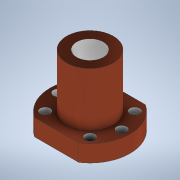
# Autodesk Inventor part: Tuerca 16
Saved by Autodesk Inventor 2021 (Build 250183000, 183)
## iProperties
Created: 2022-01-20
Part Number: Tuerca 16
Material: Generic
Document SubType Name: Modeling
Designer: deuts
Density: 1 g/cm^3
Appearance: Default
Author: deuts
Autodesk Inventor part; units mm, degrees
ref_plane "YZ Plane" through (0, 0, 0) normal (1, 0, 0) x (0, 1, 0)
ref_plane "XZ Plane" through (0, 0, 0) normal (0, 1, 0) x (-1, 0, 0)
ref_plane "XY Plane" through (0, 0, 0) normal (0, 0, 1) x (1, 0, 0)
sketch "Sketch1" plane through (0, 0, 0) normal (0, 1, 0) x (-1, 0, 0)
  line L0 (-13.2665, 20) -> (13.2665, 20)
  line L1 (13.2665, -20) -> (-13.2665, -20)
  arc A0 (13.2665, -20) -> (13.2665, 20) centre (0, 0) ccw
  arc A1 (-13.2665, 20) -> (-13.2665, -20) centre (0, 0) ccw
  circle A2 centre (19, 0) radius 3
  circle A3 centre (13.435, 13.435) radius 3
  circle A4 centre (13.435, -13.435) radius 3
  line L2 (0, 0) -> (-19, 0)
  circle A5 centre (-19, 0) radius 3
  circle A6 centre (-13.435, -13.435) radius 3
  circle A7 centre (-13.435, 13.435) radius 3
  dimension "d2" = 40
  dimension "d7" = 45
  dimension "d11" = 45
  dimension "d17" = 45
  dimension "d21" = 45
  constraints: 8 centre point, 6 end point, 4 point on circle, 2 coincident, 2 horizontal, 1 parallel, 12 other
  measures "d2" distance between parallel lines of L1 L0
extrude "Extrusion1" add sketch "Sketch1" along normal blind 10
sketch "Sketch2" plane through (0, 10, 0) normal (0, 1, 0) x (1, 0, 0)
  circle A0 centre (0, 0) radius 14
  dimension "d25" = 28
  constraints: 1 centre point, 1 coincident
  measures "d25" diameter of A0
extrude "Extrusion2" add sketch "Sketch2" along normal blind 32
sketch "Sketch3" plane through (0, 42, 0) normal (0, 1, 0) x (1, 0, 0)
  point P0 (0, 0)
  point P1 (0, 0)
  constraints: 1 coincident
hole "Hole1" at (0, 42, 0) direction (0, -1, 0) diameter 16 end through all
body "Solid1"
